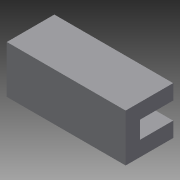
# Autodesk Inventor part: Front
Saved by Autodesk Inventor 2015 (Build 190159000, 159)
## iProperties
Created: 2015-06-23
Part Number: Front
Material: 一般
Document SubType Name: Modeling
Designer: hyt
Density: 1 g/cm^3
Appearance: 既定
Author: hyt
Autodesk Inventor part; units mm, degrees
ref_plane "YZ Plane" through (0, 0, 0) normal (1, 0, 0) x (0, 1, 0)
ref_plane "XZ Plane" through (0, 0, 0) normal (0, 1, 0) x (-1, 0, 0)
ref_plane "XY Plane" through (0, 0, 0) normal (0, 0, 1) x (1, 0, 0)
sketch "スケッチ1" plane through (0, 0, 0) normal (0, 1, 0) x (-1, 0, 0)
  line L0 (0, 0) -> (-75, 0)
  line L1 (-75, 0) -> (-75, -30)
  line L2 (-75, -30) -> (0, -30)
  line L3 (0, -30) -> (0, 0)
  dimension "d0" = 75
  dimension "d1" = 30
  constraints: 8 end point, 2 parallel, 1 horizontal, 1 perpendicular
  measures "d0" distance of L1.end L2.end
  measures "d1" distance of L2.end L0.start
extrude "押し出し1" add sketch "スケッチ1" along normal blind 30
sketch "スケッチ2" plane through (75, 0, 0) normal (1, 0, 0) x (0, 0, -1)
  line L0 (9.5, 30) -> (20.5, 30)
  line L1 (20.5, 30) -> (20.5, 9)
  line L2 (20.5, 9) -> (9.5, 9)
  line L3 (9.5, 9) -> (9.5, 30)
  line L4 (0, 30) -> (30, 30) projected
  point P0 (0, 0)
  point P1 (15, 30)
  dimension "d4" = 11
  dimension "d5" = 21
  constraints: 8 end point, 2 midpoint, 2 parallel, 1 horizontal, 1 perpendicular
  measures "d4" distance of L1.end L2.end
  measures "d5" distance of L2.end L0.start
extrude "押し出し2" cut sketch "スケッチ2" against normal blind 75
